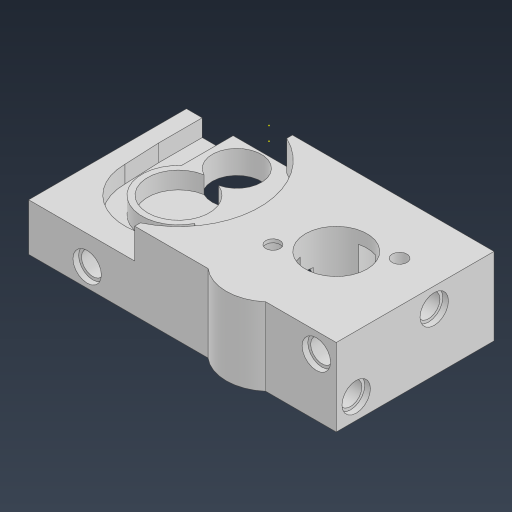
# Autodesk Inventor part: gearbox-holder-left
Saved by Autodesk Inventor 2023 (Build 270158000, 158)
## iProperties
Created: 2025-04-08
Part Number: gearbox-holder-left
Material: Generic
Document SubType Name: Modeling
Designer: szymo
Density: 1 g/cm^3
Appearance: Default
Mass: 8.72272 g
Surface Area: 68.6198 cm^2
Volume: 8.72272 cm^3
Author: szymo
Autodesk Inventor part; units mm, degrees
(part 1 of 2)
ref_plane "YZ Plane" through (0, 0, 0) normal (1, 0, 0) x (0, 1, 0)
ref_plane "XZ Plane" through (0, 0, 0) normal (0, 1, 0) x (-1, 0, 0)
ref_plane "XY Plane" through (0, 0, 0) normal (0, 0, 1) x (1, 0, 0)
ref_plane "Work Plane3" through (-21, -16.2, 14.3) normal (0, 1, 0) x (-1, 0, 0)
sketch "Sketch1" plane through (-21, -16.2, 14.3) normal (0, 1, 0) x (-1, 0, 0)
  circle A0 centre (-40.0468, 4.0664) radius 1.0564 projected
  circle A1 centre (-53.2532, -4.9664) radius 1.0564 projected
  circle A2 centre (-46.65, -0.45) radius 5 projected
  circle A3 centre (-46.65, -0.45) radius 13.85 projected
  line L0 (-23.5981, 5.436) -> (-26.6956, 8.0504) projected
  arc A4 (-26.6956, 8.0504) -> (-28.6306, 5.7578) centre (-18.95, -0.45) ccw projected
  line L1 (-28.6306, 5.7578) -> (-25.5331, 3.1435) projected
  arc A5 (-23.5981, 5.436) -> (-25.5331, 3.1435) centre (-18.95, -0.45) ccw projected
  arc A6 (-11.2044, -8.9504) -> (-9.2694, -6.6578) centre (-18.95, -0.45) ccw projected
  line L2 (-9.2694, -6.6578) -> (-12.3669, -4.0435) projected
  arc A7 (-14.3019, -6.336) -> (-12.3669, -4.0435) centre (-18.95, -0.45) ccw projected
  line L3 (-14.3019, -6.336) -> (-11.2044, -8.9504) projected
  circle A8 centre (-18.95, -0.45) radius 5 projected
  circle A9 centre (-18.95, -0.45) radius 13.85 projected
  line L4 (-25.1095, 12.4) -> (-25.1095, 13.4)
  line L5 (-25.1095, 13.4) -> (-60.5, 13.4)
  line L6 (-60.5, 13.4) -> (-60.5, -14.3)
  line L7 (-60.5, -14.3) -> (-25.1095, -14.3)
  line L8 (-25.1095, -14.3) -> (-25.1095, -13.3)
  circle A10 centre (-18.95, -0.45) radius 14.25
  circle A11 centre (-46.65, -0.45) radius 5.4
  circle A12 centre (-43.0585, 7.5289) radius 1.25 projected
  arc A13 (-39.3343, 3.3134) -> (-38.2806, 2.7608) centre (-36.6798, 7.0946) ccw projected
  arc A14 (-39.6063, 3.0878) -> (-39.3343, 3.3134) centre (-43.0585, 7.5289) ccw projected
  arc A15 (-39.2587, 1.95) -> (-39.6063, 3.0878) centre (-43.8141, 1.1803) ccw projected
  arc A16 (-39.6165, 1.7224) -> (-39.2587, 1.95) centre (-43.0585, 7.5289) ccw projected
  arc A17 (-40.4997, 2.5196) -> (-39.6165, 1.7224) centre (-36.9882, 5.5219) ccw projected
  arc A18 (-40.8192, 2.3688) -> (-40.4997, 2.5196) centre (-43.0585, 7.5289) ccw projected
  arc A19 (-40.7655, 1.1803) -> (-40.8192, 2.3688) centre (-45.3692, 1.5677) ccw projected
  arc A20 (-41.1687, 1.0489) -> (-40.7655, 1.1803) centre (-43.0585, 7.5289) ccw projected
  arc A21 (-41.8258, 2.0407) -> (-41.1687, 1.0489) centre (-37.6781, 4.0753) ccw projected
  arc A22 (-42.1729, 1.9741) -> (-41.8258, 2.0407) centre (-43.0585, 7.5289) ccw projected
  arc A23 (-42.4164, 0.8095) -> (-42.1729, 1.9741) centre (-46.7791, 2.3296) ccw projected
  arc A24 (-42.8396, 0.7825) -> (-42.4164, 0.8095) centre (-43.0585, 7.5289) ccw projected
  arc A25 (-43.2294, 1.9065) -> (-42.8396, 0.7825) centre (-38.706, 2.8458) ccw projected
  arc A26 (-43.5821, 1.9284) -> (-43.2294, 1.9065) centre (-43.0585, 7.5289) ccw projected
  arc A27 (-44.1076, 0.861) -> (-43.5821, 1.9284) centre (-47.9552, 3.4182) ccw projected
  arc A28 (-44.5242, 0.94) -> (-44.1076, 0.861) centre (-43.0585, 7.5289) ccw projected
  arc A29 (-44.6223, 2.1257) -> (-44.5242, 0.94) centre (-40.0074, 1.9105) ccw projected
  arc A30 (-44.9585, 2.2345) -> (-44.6223, 2.1257) centre (-43.0585, 7.5289) ccw projected
  arc A31 (-45.7329, 1.3314) -> (-44.9585, 2.2345) centre (-48.8237, 4.7651) ccw projected
  arc A32 (-46.1168, 1.5115) -> (-45.7329, 1.3314) centre (-43.0585, 7.5289) ccw projected
  arc A33 (-45.9169, 2.6843) -> (-46.1168, 1.5115) centre (-41.5005, 1.3282) ccw projected
  arc A34 (-46.2154, 2.8734) -> (-45.9169, 2.6843) centre (-43.0585, 7.5289) ccw projected
  arc A35 (-47.1901, 2.1912) -> (-46.2154, 2.8734) centre (-49.3299, 6.2857) ccw projected
  arc A36 (-47.5172, 2.4611) -> (-47.1901, 2.1912) centre (-43.0585, 7.5289) ccw projected
  arc A37 (-47.0319, 3.5474) -> (-47.5172, 2.4611) centre (-43.0915, 1.1356) ccw projected
  arc A38 (-47.274, 3.8048) -> (-47.0319, 3.5474) centre (-43.0585, 7.5289) ccw projected
  arc A39 (-48.3878, 3.3864) -> (-47.274, 3.8048) centre (-49.442, 7.8844) ccw projected
  arc A40 (-48.6374, 3.7292) -> (-48.3878, 3.3864) centre (-43.0585, 7.5289) ccw projected
  arc A41 (-47.8972, 4.6606) -> (-48.6374, 3.7292) centre (-44.6804, 1.3446) ccw projected
  arc A42 (-48.0678, 4.9701) -> (-47.8972, 4.6606) centre (-43.0585, 7.5289) ccw projected
  arc A43 (-49.2506, 4.8419) -> (-48.0678, 4.9701) centre (-49.1531, 9.4608) ccw projected
  arc A44 (-49.4071, 5.236) -> (-49.2506, 4.8419) centre (-43.0585, 7.5289) ccw projected
  arc A45 (-48.4585, 5.9541) -> (-49.4071, 5.236) centre (-46.1674, 1.9423) ccw projected
  arc A46 (-48.5467, 6.2963) -> (-48.4585, 5.9541) centre (-43.0585, 7.5289) ccw projected
  arc A47 (-49.7243, 6.4662) -> (-48.5467, 6.2963) centre (-48.4812, 10.9157) ccw projected
  arc A48 (-49.7779, 6.8868) -> (-49.7243, 6.4662) centre (-43.0585, 7.5289) ccw projected
  arc A49 (-48.6805, 7.3465) -> (-49.7779, 6.8868) centre (-47.4591, 2.891) ccw projected
  arc A50 (-48.6809, 7.6999) -> (-48.6805, 7.3465) centre (-43.0585, 7.5289) ccw projected
  arc A51 (-49.7792, 8.1573) -> (-48.6809, 7.6999) centre (-47.4685, 12.1579) ccw projected
  arc A52 (-49.7264, 8.5781) -> (-49.7792, 8.1573) centre (-43.0585, 7.5289) ccw projected
  arc A53 (-48.5493, 8.7504) -> (-49.7264, 8.5781) centre (-48.4743, 4.1311) ccw projected
  arc A54 (-48.4617, 9.0927) -> (-48.5493, 8.7504) centre (-43.0585, 7.5289) ccw projected
  arc A55 (-49.4117, 9.8089) -> (-48.4617, 9.0927) centre (-46.1788, 13.1092) ccw projected
  arc A56 (-49.256, 10.2034) -> (-49.4117, 9.8089) centre (-43.0585, 7.5289) ccw projected
  arc A57 (-48.073, 10.0775) -> (-49.256, 10.2034) centre (-49.1491, 5.5847) ccw projected
  arc A58 (-47.9031, 10.3873) -> (-48.073, 10.0775) centre (-43.0585, 7.5289) ccw projected
  arc A59 (-48.6451, 11.3173) -> (-47.9031, 10.3873) centre (-44.693, 13.7099) ccw projected
  arc A60 (-48.3962, 11.6606) -> (-48.6451, 11.3173) centre (-43.0585, 7.5289) ccw projected
  arc A61 (-47.2816, 11.2445) -> (-48.3962, 11.6606) centre (-49.4413, 7.1604) ccw projected
  arc A62 (-47.04, 11.5023) -> (-47.2816, 11.2445) centre (-43.0585, 7.5289) ccw projected
  arc A63 (-47.5275, 12.5876) -> (-47.04, 11.5023) centre (-43.1045, 13.9222) ccw projected
  arc A64 (-47.201, 12.8583) -> (-47.5275, 12.5876) centre (-43.0585, 7.5289) ccw projected
  arc A65 (-46.2249, 12.178) -> (-47.201, 12.8583) centre (-49.3324, 8.7593) ccw projected
  arc A66 (-45.9268, 12.3677) -> (-46.2249, 12.178) centre (-43.0585, 7.5289) ccw projected
  arc A67 (-46.129, 13.5401) -> (-45.9268, 12.3677) centre (-41.5131, 13.7328) ccw projected
  arc A68 (-45.7455, 13.721) -> (-46.129, 13.5401) centre (-43.0585, 7.5289) ccw projected
  arc A69 (-44.9693, 12.8194) -> (-45.7455, 13.721) centre (-48.8293, 10.281) ccw projected
  arc A70 (-44.6333, 12.929) -> (-44.9693, 12.8194) centre (-43.0585, 7.5289) ccw projected
  arc A71 (-44.5377, 14.1149) -> (-44.6333, 12.929) centre (-40.0188, 13.1536) ccw projected
  arc A72 (-44.1212, 14.1948) -> (-44.5377, 14.1149) centre (-43.0585, 7.5289) ccw projected
  arc A73 (-43.5935, 13.1284) -> (-44.1212, 14.1948) centre (-47.9636, 11.6296) ccw projected
  arc A74 (-43.2409, 13.151) -> (-43.5935, 13.1284) centre (-43.0585, 7.5289) ccw projected
  arc A75 (-42.8533, 14.2758) -> (-43.2409, 13.151) centre (-38.7155, 12.221) ccw projected
  arc A76 (-42.4301, 14.2496) -> (-42.8533, 14.2758) centre (-43.0585, 7.5289) ccw projected
  arc A77 (-42.1842, 13.0856) -> (-42.4301, 14.2496) centre (-46.7897, 12.7207) ccw projected
  arc A78 (-41.837, 13.0197) -> (-42.1842, 13.0856) centre (-43.0585, 7.5289) ccw projected
  arc A79 (-41.1819, 14.0128) -> (-41.837, 13.0197) centre (-37.6851, 10.9935) ccw projected
  arc A80 (-40.7785, 13.8822) -> (-41.1819, 14.0128) centre (-43.0585, 7.5289) ccw projected
  arc A81 (-40.8298, 12.6936) -> (-40.7785, 13.8822) centre (-45.3813, 13.4855) ccw projected
  arc A82 (-40.5099, 12.5435) -> (-40.8298, 12.6936) centre (-43.0585, 7.5289) ccw projected
  arc A83 (-39.6284, 13.3424) -> (-40.5099, 12.5435) centre (-36.9923, 9.5484) ccw projected
  arc A84 (-39.2701, 13.1156) -> (-39.6284, 13.3424) centre (-43.0585, 7.5289) ccw projected
  arc A85 (-39.6154, 11.9771) -> (-39.2701, 13.1156) centre (-43.827, 13.876) ccw projected
  arc A86 (-39.3429, 11.7521) -> (-39.6154, 11.9771) centre (-43.0585, 7.5289) ccw projected
  arc A87 (-38.2904, 12.3068) -> (-39.3429, 11.7521) centre (-36.6807, 7.9763) ccw projected
  arc A88 (-37.9998, 11.998) -> (-38.2904, 12.3068) centre (-43.0585, 7.5289) ccw projected
  arc A89 (-38.6174, 10.9811) -> (-37.9998, 11.998) centre (-42.2244, 13.8678) ccw projected
  arc A90 (-38.4094, 10.6954) -> (-38.6174, 10.9811) centre (-43.0585, 7.5289) ccw projected
  arc A91 (-37.252, 10.9709) -> (-38.4094, 10.6954) centre (-36.7698, 6.3762) ccw projected
  arc A92 (-37.0473, 10.5995) -> (-37.252, 10.9709) centre (-43.0585, 7.5289) ccw projected
  arc A93 (-37.8984, 9.7682) -> (-37.0473, 10.5995) centre (-40.6742, 13.4612) ccw projected
  arc A94 (-37.768, 9.4397) -> (-37.8984, 9.7682) centre (-43.0585, 7.5289) ccw projected
  arc A95 (-36.5784, 9.4187) -> (-37.768, 9.4397) centre (-37.254, 4.8485) ccw projected
  arc A96 (-36.4725, 9.0081) -> (-36.5784, 9.4187) centre (-43.0585, 7.5289) ccw projected
  arc A97 (-37.5036, 8.4146) -> (-36.4725, 9.0081) centre (-39.2738, 12.6819) ccw projected
  arc A98 (-37.459, 8.064) -> (-37.5036, 8.4146) centre (-43.0585, 7.5289) ccw projected
  arc A99 (-36.312, 7.7478) -> (-37.459, 8.064) centre (-38.103, 3.4892) ccw projected
  arc A100 (-36.3116, 7.3238) -> (-36.312, 7.7478) centre (-43.0585, 7.5289) ccw projected
  arc A101 (-37.4579, 7.0053) -> (-36.3116, 7.3238) centre (-38.1113, 11.5788) ccw projected
  arc A102 (-37.5018, 6.6547) -> (-37.4579, 7.0053) centre (-43.0585, 7.5289) ccw projected
  arc A103 (-36.4695, 6.0632) -> (-37.5018, 6.6547) centre (-39.2633, 2.3837) ccw projected
  arc A104 (-36.5746, 5.6524) -> (-36.4695, 6.0632) centre (-43.0585, 7.5289) ccw projected
  arc A105 (-37.7641, 5.6289) -> (-36.5746, 5.6524) centre (-37.2595, 10.2212) ccw projected
  arc A106 (-37.8938, 5.3003) -> (-37.7641, 5.6289) centre (-43.0585, 7.5289) ccw projected
  arc A107 (-37.0411, 4.4706) -> (-37.8938, 5.3003) centre (-40.6621, 1.6016) ccw projected
  arc A108 (-37.245, 4.0988) -> (-37.0411, 4.4706) centre (-43.0585, 7.5289) ccw projected
  arc A109 (-38.4029, 4.372) -> (-37.245, 4.0988) centre (-36.7722, 8.6945) ccw projected
  arc A110 (-38.6103, 4.0859) -> (-38.4029, 4.372) centre (-43.0585, 7.5289) ccw projected
  arc A111 (-37.9907, 3.0703) -> (-38.6103, 4.0859) centre (-42.2115, 1.1918) ccw projected
  arc A112 (-38.2806, 2.7608) -> (-37.9907, 3.0703) centre (-43.0585, 7.5289) ccw projected
  circle A113 centre (-43.0585, 7.5289) radius 6.75
  circle A114 centre (-43.0585, 7.5289) radius 7.15
  circle A115 centre (-43.0585, 7.5289) radius 7.75
  point P0 (-21, -14.3)
  point P1 (-37.9995, 13.4)
  point P2 (-48.1174, 13.4)
  dimension "d2" = 0.4
  dimension "d3" = 1
  dimension "d5" = 1
  dimension "d6" = 0.4
  dimension "d13" = 0.4
  dimension "d14" = 0.6
  constraints: 10 end point, 4 centre point, 4 perpendicular, 3 tangent, 2 point on circle, 1 coincident, 1 vertical, 3 other
  measures "d2" radial gap between concentric circles of A9 A10
  measures "d3" distance of L7.end L8.end
  measures "d5" distance of L4.start L4.end
  measures "d6" radial gap between concentric circles of A2 A11
  measures "d14" radial gap between concentric circles of A114 A115
extrude "Extrusion1" add sketch "Sketch1" against normal blind 3.1 contours A0 A13 A14 | A0 A14 A15 A16 A17 A18 A19 A20 A21 A22 A11 A42 A43 A44 A45 A46 A47 A48 A49 A50 A51 A52 A53 A54 A55 A56 A57 A58 A59 A60 A61 A62 A63 A64 A65 A66 A67 A3 A69 A70 A71 A93 A94 A95 A97 A98 A99 A100 A101 A102 A103 A104 A105 A106 A107 A108 A109 A110 A111 A112 A13 | A14 A13 A0 | A0 A13 A113 A15 A14 | A112 A113 A108 A104 A100 A3 A114 A11 A20 A16 | A111 A110 A109 A113 | A113 A19 A18 A17 | A107 A106 A105 A113 | A113 A11 A22 A21 | A103 A102 A101 A113 | A114 A3 A115 A11 | A11 A113 A43 A42 | A115 A3 A10 A11 | A11 A114 A3 A113 A64 A60 A56 A52 A48 A44 | A115 L5 L4 A10 A3 | A3 A114 L5 A115 | A3 A113 A96 A92 A88 A84 L5 A114 | A99 A98 A97 A3 A113 | A11 A115 A3 A114 | A3 A97 A113 | A114 L5 A115 | L5 A113 A80 A76 A72 A68 A3 A114 | A114 L5 A3 | A3 A115 L5 A114 | A113 A47 A46 A45 | A3 L6 L5 A115 | A10 L8 L7 A3 | A3 A95 A96 A97 | A113 A83 A82 A81 L5 | L5 A81 A113 | A3 L7 L6 | A95 A94 A93 A3 | A3 A93 A113 A95 | A81 A82 A83 A84 A85 A86 A87 A88 A89 A90 A91 A92 A93 A3 A71 L5 A73 A74 A75 A77 A78 A79 | L5 A79 A80 A81 | L5 A67 A3 | A113 A67 L5 | A3 A67 A66 A65 A113 | A113 A51 A50 A49 | A79 A78 A77 L5 | L5 A77 A113 A79 | A113 A87 A86 A85 | A67 L5 A69 A3 | A67 A68 A69 L5 | A71 A70 A69 A3 | A3 A69 L5 A71 | A91 A90 A89 A113 | L5 A75 A76 A77 | A69 A113 A71 L5 | A63 A62 A61 A113 | A113 A55 A54 A53 | A71 A72 A73 L5 | A75 A74 A73 L5 | L5 A73 A113 A75 | A59 A58 A57 A113 | A1 | A12
sketch "Sketch2" plane through (-21, -19.3, 14.3) normal (0, -1, 0) x (1, 0, 0)
  circle A0 centre (43.0585, 7.5289) radius 1.25 projected
  arc A1 (38.2806, 2.7608) -> (39.3343, 3.3134) centre (36.6798, 7.0946) ccw projected
  arc A2 (39.3343, 3.3134) -> (39.6063, 3.0878) centre (43.0585, 7.5289) ccw projected
  arc A3 (39.6063, 3.0878) -> (39.2587, 1.95) centre (43.8141, 1.1803) ccw projected
  arc A4 (39.2587, 1.95) -> (39.6165, 1.7224) centre (43.0585, 7.5289) ccw projected
  arc A5 (39.6165, 1.7224) -> (40.4997, 2.5196) centre (36.9882, 5.5219) ccw projected
  arc A6 (40.4997, 2.5196) -> (40.8192, 2.3688) centre (43.0585, 7.5289) ccw projected
  arc A7 (40.8192, 2.3688) -> (40.7655, 1.1803) centre (45.3692, 1.5677) ccw projected
  arc A8 (40.7655, 1.1803) -> (41.1687, 1.0489) centre (43.0585, 7.5289) ccw projected
  arc A9 (41.1687, 1.0489) -> (41.8258, 2.0407) centre (37.6781, 4.0753) ccw projected
  arc A10 (41.8258, 2.0407) -> (42.1729, 1.9741) centre (43.0585, 7.5289) ccw projected
  arc A11 (42.1729, 1.9741) -> (42.4164, 0.8095) centre (46.7791, 2.3296) ccw projected
  arc A12 (42.4164, 0.8095) -> (42.8396, 0.7825) centre (43.0585, 7.5289) ccw projected
  arc A13 (42.8396, 0.7825) -> (43.2294, 1.9065) centre (38.706, 2.8458) ccw projected
  arc A14 (43.2294, 1.9065) -> (43.5821, 1.9284) centre (43.0585, 7.5289) ccw projected
  arc A15 (43.5821, 1.9284) -> (44.1076, 0.861) centre (47.9552, 3.4182) ccw projected
  arc A16 (44.1076, 0.861) -> (44.5242, 0.94) centre (43.0585, 7.5289) ccw projected
  arc A17 (44.5242, 0.94) -> (44.6223, 2.1257) centre (40.0074, 1.9105) ccw projected
  arc A18 (44.6223, 2.1257) -> (44.9585, 2.2345) centre (43.0585, 7.5289) ccw projected
  arc A19 (44.9585, 2.2345) -> (45.7329, 1.3314) centre (48.8237, 4.7651) ccw projected
  arc A20 (45.7329, 1.3314) -> (46.1168, 1.5115) centre (43.0585, 7.5289) ccw projected
  arc A21 (46.1168, 1.5115) -> (45.9169, 2.6843) centre (41.5005, 1.3282) ccw projected
  arc A22 (45.9169, 2.6843) -> (46.2154, 2.8734) centre (43.0585, 7.5289) ccw projected
  arc A23 (46.2154, 2.8734) -> (47.1901, 2.1912) centre (49.3299, 6.2857) ccw projected
  arc A24 (47.1901, 2.1912) -> (47.5172, 2.4611) centre (43.0585, 7.5289) ccw projected
  arc A25 (47.5172, 2.4611) -> (47.0319, 3.5474) centre (43.0915, 1.1356) ccw projected
  arc A26 (47.0319, 3.5474) -> (47.274, 3.8048) centre (43.0585, 7.5289) ccw projected
  arc A27 (47.274, 3.8048) -> (48.3878, 3.3864) centre (49.442, 7.8844) ccw projected
  arc A28 (48.3878, 3.3864) -> (48.6374, 3.7292) centre (43.0585, 7.5289) ccw projected
  arc A29 (48.6374, 3.7292) -> (47.8972, 4.6606) centre (44.6804, 1.3446) ccw projected
  arc A30 (47.8972, 4.6606) -> (48.0678, 4.9701) centre (43.0585, 7.5289) ccw projected
  arc A31 (48.0678, 4.9701) -> (49.2506, 4.8419) centre (49.1531, 9.4608) ccw projected
  arc A32 (49.2506, 4.8419) -> (49.4071, 5.236) centre (43.0585, 7.5289) ccw projected
  arc A33 (49.4071, 5.236) -> (48.4585, 5.9541) centre (46.1674, 1.9423) ccw projected
  arc A34 (48.4585, 5.9541) -> (48.5467, 6.2963) centre (43.0585, 7.5289) ccw projected
  arc A35 (48.5467, 6.2963) -> (49.7243, 6.4662) centre (48.4812, 10.9157) ccw projected
  arc A36 (49.7243, 6.4662) -> (49.7779, 6.8868) centre (43.0585, 7.5289) ccw projected
  arc A37 (49.7779, 6.8868) -> (48.6805, 7.3465) centre (47.4591, 2.891) ccw projected
  arc A38 (48.6805, 7.3465) -> (48.6809, 7.6999) centre (43.0585, 7.5289) ccw projected
  arc A39 (48.6809, 7.6999) -> (49.7792, 8.1573) centre (47.4685, 12.1579) ccw projected
  arc A40 (49.7792, 8.1573) -> (49.7264, 8.5781) centre (43.0585, 7.5289) ccw projected
  arc A41 (49.7264, 8.5781) -> (48.5493, 8.7504) centre (48.4743, 4.1311) ccw projected
  arc A42 (48.5493, 8.7504) -> (48.4617, 9.0927) centre (43.0585, 7.5289) ccw projected
  arc A43 (48.4617, 9.0927) -> (49.4117, 9.8089) centre (46.1788, 13.1092) ccw projected
  arc A44 (49.4117, 9.8089) -> (49.256, 10.2034) centre (43.0585, 7.5289) ccw projected
  arc A45 (49.256, 10.2034) -> (48.073, 10.0775) centre (49.1491, 5.5847) ccw projected
  arc A46 (48.073, 10.0775) -> (47.9031, 10.3873) centre (43.0585, 7.5289) ccw projected
  arc A47 (47.9031, 10.3873) -> (48.6451, 11.3173) centre (44.693, 13.7099) ccw projected
  arc A48 (48.6451, 11.3173) -> (48.3962, 11.6606) centre (43.0585, 7.5289) ccw projected
  arc A49 (48.3962, 11.6606) -> (47.2816, 11.2445) centre (49.4413, 7.1604) ccw projected
  arc A50 (47.2816, 11.2445) -> (47.04, 11.5023) centre (43.0585, 7.5289) ccw projected
  arc A51 (47.04, 11.5023) -> (47.5275, 12.5876) centre (43.1045, 13.9222) ccw projected
  arc A52 (47.5275, 12.5876) -> (47.201, 12.8583) centre (43.0585, 7.5289) ccw projected
  arc A53 (47.201, 12.8583) -> (46.2249, 12.178) centre (49.3324, 8.7593) ccw projected
  arc A54 (46.2249, 12.178) -> (45.9268, 12.3677) centre (43.0585, 7.5289) ccw projected
  arc A55 (45.9268, 12.3677) -> (46.129, 13.5401) centre (41.5131, 13.7328) ccw projected
  arc A56 (46.129, 13.5401) -> (45.7455, 13.721) centre (43.0585, 7.5289) ccw projected
  arc A57 (45.7455, 13.721) -> (44.9693, 12.8194) centre (48.8293, 10.281) ccw projected
  arc A58 (44.9693, 12.8194) -> (44.6333, 12.929) centre (43.0585, 7.5289) ccw projected
  arc A59 (44.6333, 12.929) -> (44.5377, 14.1149) centre (40.0188, 13.1536) ccw projected
  arc A60 (44.5377, 14.1149) -> (44.1212, 14.1948) centre (43.0585, 7.5289) ccw projected
  arc A61 (44.1212, 14.1948) -> (43.5935, 13.1284) centre (47.9636, 11.6296) ccw projected
  arc A62 (43.5935, 13.1284) -> (43.2409, 13.151) centre (43.0585, 7.5289) ccw projected
  arc A63 (43.2409, 13.151) -> (42.8533, 14.2758) centre (38.7155, 12.221) ccw projected
  arc A64 (42.8533, 14.2758) -> (42.4301, 14.2496) centre (43.0585, 7.5289) ccw projected
  arc A65 (42.4301, 14.2496) -> (42.1842, 13.0856) centre (46.7897, 12.7207) ccw projected
  arc A66 (42.1842, 13.0856) -> (41.837, 13.0197) centre (43.0585, 7.5289) ccw projected
  arc A67 (41.837, 13.0197) -> (41.1819, 14.0128) centre (37.6851, 10.9935) ccw projected
  arc A68 (41.1819, 14.0128) -> (40.7785, 13.8822) centre (43.0585, 7.5289) ccw projected
  arc A69 (40.7785, 13.8822) -> (40.8298, 12.6936) centre (45.3813, 13.4855) ccw projected
  arc A70 (40.8298, 12.6936) -> (40.5099, 12.5435) centre (43.0585, 7.5289) ccw projected
  arc A71 (40.5099, 12.5435) -> (39.6284, 13.3424) centre (36.9923, 9.5484) ccw projected
  arc A72 (39.6284, 13.3424) -> (39.2701, 13.1156) centre (43.0585, 7.5289) ccw projected
  arc A73 (39.2701, 13.1156) -> (39.6154, 11.9771) centre (43.827, 13.876) ccw projected
  arc A74 (39.6154, 11.9771) -> (39.3429, 11.7521) centre (43.0585, 7.5289) ccw projected
  arc A75 (39.3429, 11.7521) -> (38.2904, 12.3068) centre (36.6807, 7.9763) ccw projected
  arc A76 (38.2904, 12.3068) -> (37.9998, 11.998) centre (43.0585, 7.5289) ccw projected
  arc A77 (37.9998, 11.998) -> (38.6174, 10.9811) centre (42.2244, 13.8678) ccw projected
  arc A78 (38.6174, 10.9811) -> (38.4094, 10.6954) centre (43.0585, 7.5289) ccw projected
  arc A79 (38.4094, 10.6954) -> (37.252, 10.9709) centre (36.7698, 6.3762) ccw projected
  arc A80 (37.252, 10.9709) -> (37.0473, 10.5995) centre (43.0585, 7.5289) ccw projected
  arc A81 (37.0473, 10.5995) -> (37.8984, 9.7682) centre (40.6742, 13.4612) ccw projected
  arc A82 (37.8984, 9.7682) -> (37.768, 9.4397) centre (43.0585, 7.5289) ccw projected
  arc A83 (37.768, 9.4397) -> (36.5784, 9.4187) centre (37.254, 4.8485) ccw projected
  arc A84 (36.5784, 9.4187) -> (36.4725, 9.0081) centre (43.0585, 7.5289) ccw projected
  arc A85 (36.4725, 9.0081) -> (37.5036, 8.4146) centre (39.2738, 12.6819) ccw projected
  arc A86 (37.5036, 8.4146) -> (37.459, 8.064) centre (43.0585, 7.5289) ccw projected
  arc A87 (37.459, 8.064) -> (36.312, 7.7478) centre (38.103, 3.4892) ccw projected
  arc A88 (36.312, 7.7478) -> (36.3116, 7.3238) centre (43.0585, 7.5289) ccw projected
  arc A89 (36.3116, 7.3238) -> (37.4579, 7.0053) centre (38.1113, 11.5788) ccw projected
  arc A90 (37.4579, 7.0053) -> (37.5018, 6.6547) centre (43.0585, 7.5289) ccw projected
  arc A91 (37.5018, 6.6547) -> (36.4695, 6.0632) centre (39.2633, 2.3837) ccw projected
  arc A92 (36.4695, 6.0632) -> (36.5746, 5.6524) centre (43.0585, 7.5289) ccw projected
  arc A93 (36.5746, 5.6524) -> (37.7641, 5.6289) centre (37.2595, 10.2212) ccw projected
  arc A94 (37.7641, 5.6289) -> (37.8938, 5.3003) centre (43.0585, 7.5289) ccw projected
  arc A95 (37.8938, 5.3003) -> (37.0411, 4.4706) centre (40.6621, 1.6016) ccw projected
  arc A96 (37.0411, 4.4706) -> (37.245, 4.0988) centre (43.0585, 7.5289) ccw projected
  arc A97 (37.245, 4.0988) -> (38.4029, 4.372) centre (36.7722, 8.6945) ccw projected
  arc A98 (38.4029, 4.372) -> (38.6103, 4.0859) centre (43.0585, 7.5289) ccw projected
  arc A99 (38.6103, 4.0859) -> (37.9907, 3.0703) centre (42.2115, 1.1918) ccw projected
  arc A100 (37.9907, 3.0703) -> (38.2806, 2.7608) centre (43.0585, 7.5289) ccw projected
  circle A101 centre (43.0585, 7.5289) radius 6.75
  circle A102 centre (43.0585, 7.5289) radius 7.15
  circle A103 centre (43.0585, 7.5289) radius 7.75
  line L0 (25.1095, 13.4) -> (25.1095, 12.4) projected
  arc A104 (25.1095, -13.3) -> (25.1095, 12.4) centre (18.95, -0.45) ccw projected
  line L1 (25.1095, -13.3) -> (25.1095, -14.3) projected
  line L2 (25.1095, -14.3) -> (60.5, -14.3) projected
  line L3 (60.5, -14.3) -> (60.5, 13.4) projected
  line L4 (60.5, 13.4) -> (48.1174, 13.4) projected
  circle A105 centre (46.65, -0.45) radius 5.4 projected
  arc A106 (48.1174, 13.4) -> (37.9995, 13.4) centre (43.0585, 7.5289) ccw projected
  line L5 (37.9995, 13.4) -> (25.1095, 13.4) projected
  point P0 (21, -14.3)
  point P1 (49.3884, 4.2041)
  point P2 (41.3503, 0.586)
  point P3 (37.8284, 13.4)
  point P4 (37.9995, 13.4)
  dimension "d9" = 0.4
  dimension "d10" = 0.6
  constraints: 2 centre point, 1 coincident, 3 other
  measures "d10" radial gap between concentric circles of A102 A103
extrude "Extrusion2" add sketch "Sketch2" along normal blind 2.2 contours A105 A103 A102 | A105 A103 L4 L3 L2 L1 A104 L0 L5 picked at (47.797, 13.0993)
sketch "Sketch3" plane through (-21, -21.5, 14.3) normal (0, -1, 0) x (1, 0, 0)
  line L0 (37.9995, 13.4) -> (25.1095, 13.4) projected
  line L1 (25.1095, 13.4) -> (25.1095, 12.4) projected
  arc A0 (25.1095, -13.3) -> (25.1095, 12.4) centre (18.95, -0.45) ccw projected
  line L2 (25.1095, -13.3) -> (25.1095, -14.3) projected
  line L3 (25.1095, -14.3) -> (60.5, -14.3) projected
  line L4 (60.5, -14.3) -> (60.5, 13.4) projected
  line L5 (60.5, 13.4) -> (48.1174, 13.4) projected
  arc A1 (48.1174, 13.4) -> (37.9995, 13.4) centre (43.0585, 7.5289) ccw projected
  arc A2 (49.3884, 4.2041) -> (41.3503, 0.586) centre (43.0585, 7.5289) ccw projected
  arc A3 (41.3503, 0.586) -> (49.3884, 4.2041) centre (46.65, -0.45) ccw projected
  circle A4 centre (20, -9.6433) radius 12.5 projected
  line L6 (25.1095, 12.4) -> (25.1095, 13.4) projected
  line L7 (25.1095, 13.4) -> (13.5564, 13.4)
  line L8 (13.5564, 13.4) -> (6.5, 13.4)
  line L9 (6.5, 13.4) -> (6.5, -14.3)
  line L10 (25.1095, -14.3) -> (25.1095, -13.3) projected
  line L11 (6.5, -14.3) -> (25.1095, -14.3)
  line L12 (6.5, 13.4) -> (12.5, 13.4)
  line L13 (12.5, 13.4) -> (12.5, 7.4)
  line L14 (12.5, 7.4) -> (6.5, 7.4)
  line L15 (6.5, 7.4) -> (6.5, 13.4)
  circle A5 centre (18.95, -0.45) radius 5.4
  circle A6 centre (18.95, -0.45) radius 6.4
  circle A7 centre (20, -9.6433) radius 4 projected
  circle A8 centre (20, -9.6433) radius 4.3
  circle A9 centre (20, -9.6433) radius 5.3
  line L16 (23.5981, 5.436) -> (26.6956, 8.0504) projected
  arc A10 (28.6306, 5.7578) -> (26.6956, 8.0504) centre (18.95, -0.45) ccw projected
  line L17 (28.6306, 5.7578) -> (25.5331, 3.1435) projected
  arc A11 (25.5331, 3.1435) -> (23.5981, 5.436) centre (18.95, -0.45) ccw projected
  arc A12 (9.2694, -6.6578) -> (11.2044, -8.9504) centre (18.95, -0.45) ccw projected
  line L18 (9.2694, -6.6578) -> (12.3669, -4.0435) projected
  arc A13 (12.3669, -4.0435) -> (14.3019, -6.336) centre (18.95, -0.45) ccw projected
  line L19 (14.3019, -6.336) -> (11.2044, -8.9504) projected
  circle A14 centre (18.95, -0.45) radius 5 projected
  circle A15 centre (18.95, -0.45) radius 13.85 projected
  line L20 (14.7, -5.2351) -> (14.7, -14.3)
  line L21 (9.2694, -6.6578) -> (9.2694, -14.3)
  circle A16 centre (18.95, -0.45) radius 9.4
  line L22 (26.6956, 8.0504) -> (20.7823, 8.7697)
  line L23 (9.55, -0.45) -> (9.2694, -6.6578)
  line L24 (25.5331, 3.1435) -> (24.6721, 2.4167)
  point P0 (21, -14.3)
  point P1 (15.3858, -7.0359)
  point P2 (12.5, 13.4)
  point P3 (13.1701, -14.3)
  point P4 (8.7954, -14.3)
  point P5 (20.9759, -5.4556)
  point P6 (18.1049, -5.7835)
  dimension "d16" = 6
  dimension "d17" = 6
  dimension "d18" = 13.5
  dimension "d34" = 1
  dimension "d37" = 0.3
  dimension "d141" = 1
  dimension "d142" = 0.4
  dimension "d144" = 3
  constraints: 26 end point, 5 perpendicular, 4 centre point, 4 point on circle, 4 point on line, 2 coincident, 2 collinear, 2 horizontal, 2 parallel, 1 vertical, 3 other
  measures "d16" distance of L13.end L14.end
  measures "d17" distance of L12.end L13.end
  measures "d18" distance from line of L9 A4.centre
  measures "d34" radial gap between concentric circles of A5 A6
  measures "d37" radial gap between concentric circles of A7 A8
  measures "d142" radial gap between concentric circles of A5 A14
  measures "d144" radial gap between concentric circles of A6 A16
extrude "Extrusion3" add sketch "Sketch3" along normal blind 0.4 contours A1 L5 L4 L3 A4 A0 L1 L0 | L1 A0 A4 A15 L7 | A15 L13 L8 L7 | A15 A4 A16 L17 A10 L22 L23 L9 L14 L13 | A4 L3 L2 A0 | A0 L2 L11 A9 A15 A4 | A15 L14 L9 L8 L13 | L13 L14 A15 | A15 A9 A16 A4 | A15 L9 L14 | A16 A9 A6 A4 | A4 A6 L24 L17 A16 | A15 A9 A16 A8 | A9 L11 A15 | L11 L9 A15 A4 | A4 A15 L21 L11 | A6 A9 A5 A4 | A4 A5 A6 | L11 A9 A15 | A4 L23 L21 A15 | L11 L20 A15 A9 | A16 A8 A6 A9 | A15 L20 A9 | A5 A9 A6 A4 | A6 A8 A5 A9 | L20 A16 A9 | A5 A8 A6 A9 | A6 A9 A16 L20 | A9 A6 A8 A16
sketch "Sketch4" plane through (-21, -21.9, 14.3) normal (0, -1, 0) x (1, 0, 0)
  circle A0 centre (35.7557, 2.709) radius 1.25 projected
  arc A1 (29.263, 4.5551) -> (30.2592, 3.9047) centre (32.2659, 8.066) ccw projected
  arc A2 (30.2592, 3.9047) -> (30.195, 3.5572) centre (35.7557, 2.709) ccw projected
  arc A3 (30.195, 3.5572) -> (29.0321, 3.3058) centre (30.5815, -1.0466) ccw projected
  arc A4 (29.0321, 3.3058) -> (29.0079, 2.8825) centre (35.7557, 2.709) ccw projected
  arc A5 (29.0079, 2.8825) -> (30.1346, 2.5002) centre (31.0433, 7.0299) ccw projected
  arc A6 (30.1346, 2.5002) -> (30.1588, 2.1476) centre (35.7557, 2.709) ccw projected
  arc A7 (30.1588, 2.1476) -> (29.0949, 1.615) centre (31.678, -2.2153) ccw projected
  arc A8 (29.0949, 1.615) -> (29.1768, 1.1989) centre (35.7557, 2.709) ccw projected
  arc A9 (29.1768, 1.1989) -> (30.3631, 1.1088) centre (30.1168, 5.7222) ccw projected
  arc A10 (30.3631, 1.1088) -> (30.4742, 0.7734) centre (35.7557, 2.709) ccw projected
  arc A11 (30.4742, 0.7734) -> (29.5763, -0.0071) centre (33.0308, -3.0747) ccw projected
  arc A12 (29.5763, -0.0071) -> (29.759, -0.3898) centre (35.7557, 2.709) ccw projected
  arc A13 (29.759, -0.3898) -> (30.9304, -0.182) centre (29.5446, 4.2252) ccw projected
  arc A14 (30.9304, -0.182) -> (31.1215, -0.4793) centre (35.7557, 2.709) ccw projected
  arc A15 (31.1215, -0.4793) -> (30.4459, -1.4585) centre (34.5547, -3.5706) ccw projected
  arc A16 (30.4459, -1.4585) -> (30.718, -1.7837) centre (35.7557, 2.709) ccw projected
  arc A17 (30.718, -1.7837) -> (31.801, -1.2911) centre (29.3627, 2.6329) ccw projected
  arc A18 (31.801, -1.2911) -> (32.06, -1.5316) centre (35.7557, 2.709) ccw projected
  arc A19 (32.06, -1.5316) -> (31.6491, -2.6481) centre (36.1542, -3.672) ccw projected
  arc A20 (31.6491, -2.6481) -> (31.9936, -2.8954) centre (35.7557, 2.709) ccw projected
  arc A21 (31.9936, -2.8954) -> (32.92, -2.149) centre (29.5824, 1.0455) ccw projected
  arc A22 (32.92, -2.149) -> (33.2307, -2.3174) centre (35.7557, 2.709) ccw projected
  arc A23 (33.2307, -2.3174) -> (33.1104, -3.5011) centre (37.7285, -3.3724) ccw projected
  arc A24 (33.1104, -3.5011) -> (33.5055, -3.6549) centre (35.7557, 2.709) ccw projected
  arc A25 (33.5055, -3.6549) -> (34.2173, -2.7015) centre (30.1901, -0.4375) ccw projected
  arc A26 (34.2173, -2.7015) -> (34.56, -2.7874) centre (35.7557, 2.709) ccw projected
  arc A27 (34.56, -2.7874) -> (34.7379, -3.9638) centre (39.1789, -2.6908) ccw projected
  arc A28 (34.7379, -3.9638) -> (35.1589, -4.0146) centre (35.7557, 2.709) ccw projected
  arc A29 (35.1589, -4.0146) -> (35.6111, -2.9141) centre (31.1475, -1.7228) ccw projected
  arc A30 (35.6111, -2.9141) -> (35.9645, -2.9121) centre (35.7557, 2.709) ccw projected
  arc A31 (35.9645, -2.9121) -> (36.4293, -4.0073) centre (40.4143, -1.6698) ccw projected
  arc A32 (36.4293, -4.0073) -> (36.8497, -3.9517) centre (35.7557, 2.709) ccw projected
  arc A33 (36.8497, -3.9517) -> (37.0141, -2.7734) centre (32.3944, -2.7295) ccw projected
  arc A34 (37.0141, -2.7734) -> (37.3559, -2.6836) centre (35.7557, 2.709) ccw projected
  arc A35 (37.3559, -2.6836) -> (38.0784, -3.6288) centre (41.3569, -0.3737) ccw projected
  arc A36 (38.0784, -3.6288) -> (38.4718, -3.4704) centre (35.7557, 2.709) ccw projected
  arc A37 (38.4718, -3.4704) -> (38.338, -2.2882) centre (33.8525, -3.3946) ccw projected
  arc A38 (38.338, -2.2882) -> (38.6467, -2.1162) centre (35.7557, 2.709) ccw projected
  arc A39 (38.6467, -2.1162) -> (39.5816, -2.852) centre (41.9475, 1.1161) ccw projected
  arc A40 (39.5816, -2.852) -> (39.9232, -2.6008) centre (35.7557, 2.709) ccw projected
  arc A41 (39.9232, -2.6008) -> (39.4996, -1.489) centre (35.4302, -3.6761) ccw projected
  arc A42 (39.4996, -1.489) -> (39.7558, -1.2457) centre (35.7557, 2.709) ccw projected
  arc A43 (39.7558, -1.2457) -> (40.8444, -1.7258) centre (42.1491, 2.706) ccw projected
  arc A44 (40.8444, -1.7258) -> (41.1128, -1.3976) centre (35.7557, 2.709) ccw projected
  arc A45 (41.1128, -1.3976) -> (40.426, -0.4261) centre (37.0283, -3.5565) ccw projected
  arc A46 (40.426, -0.4261) -> (40.6136, -0.1266) centre (35.7557, 2.709) ccw projected
  arc A47 (40.6136, -0.1266) -> (41.7874, -0.321) centre (41.949, 4.2961) ccw projected
  arc A48 (41.7874, -0.321) -> (41.9657, 0.0637) centre (35.7557, 2.709) ccw projected
  arc A49 (41.9657, 0.0637) -> (41.0589, 0.8339) centre (38.5465, -3.0432) ccw projected
  arc A50 (41.0589, 0.8339) -> (41.1662, 1.1706) centre (35.7557, 2.709) ccw projected
  arc A51 (41.1662, 1.1706) -> (42.3514, 1.2742) centre (41.3597, 5.7865) ccw projected
  arc A52 (42.3514, 1.2742) -> (42.4285, 1.6912) centre (35.7557, 2.709) ccw projected
  arc A53 (42.4285, 1.6912) -> (41.3586, 2.2117) centre (39.8893, -2.1684) ccw projected
  arc A54 (41.3586, 2.2117) -> (41.3788, 2.5645) centre (35.7557, 2.709) ccw projected
  arc A55 (41.3788, 2.5645) -> (42.501, 2.9596) centre (40.4183, 7.0835) ccw projected
  arc A56 (42.501, 2.9596) -> (42.472, 3.3827) centre (35.7557, 2.709) ccw projected
  arc A57 (42.472, 3.3827) -> (41.3063, 3.6207) centre (40.9724, -0.9872) ccw projected
  arc A58 (41.3063, 3.6207) -> (41.2381, 3.9674) centre (35.7557, 2.709) ccw projected
  arc A59 (41.2381, 3.9674) -> (42.2268, 4.6292) centre (39.184, 8.1056) ccw projected
  arc A60 (42.2268, 4.6292) -> (42.0934, 5.0318) centre (35.7557, 2.709) ccw projected
  arc A61 (42.0934, 5.0318) -> (40.9052, 4.9724) centre (41.7277, 0.4263) ccw projected
  arc A62 (40.9052, 4.9724) -> (40.7529, 5.2913) centre (35.7557, 2.709) ccw projected
  arc A63 (40.7529, 5.2913) -> (41.5459, 6.1782) centre (37.7342, 8.7886) ccw projected
  arc A64 (41.5459, 6.1782) -> (41.3167, 6.5349) centre (35.7557, 2.709) ccw projected
  arc A65 (41.3167, 6.5349) -> (40.1805, 6.182) centre (42.1078, 1.9832) ccw projected
  arc A66 (40.1805, 6.182) -> (39.9537, 6.453) centre (35.7557, 2.709) ccw projected
  arc A67 (39.9537, 6.453) -> (40.5013, 7.5092) centre (36.1601, 9.0897) ccw projected
  arc A68 (40.5013, 7.5092) -> (40.1905, 7.7977) centre (35.7557, 2.709) ccw projected
  arc A69 (40.1905, 7.7977) -> (39.1778, 7.1733) centre (42.0887, 3.5857) ccw projected
  arc A70 (39.1778, 7.1733) -> (38.8907, 7.3793) centre (35.7557, 2.709) ccw projected
  arc A71 (38.8907, 7.3793) -> (39.1584, 8.5386) centre (34.5606, 8.9898) ccw projected
  arc A72 (39.1584, 8.5386) -> (38.7857, 8.7407) centre (35.7557, 2.709) ccw projected
  arc A73 (38.7857, 8.7407) -> (37.9601, 7.8841) centre (41.6717, 5.1332) ccw projected
  arc A74 (37.9601, 7.8841) -> (37.6308, 8.0123) centre (35.7557, 2.709) ccw projected
  arc A75 (37.6308, 8.0123) -> (37.6018, 9.2017) centre (33.0362, 8.4952) ccw projected
  arc A76 (37.6018, 9.2017) -> (37.1905, 9.3048) centre (35.7557, 2.709) ccw projected
  arc A77 (37.1905, 9.3048) -> (36.6038, 8.2697) centre (40.883, 6.5283) ccw projected
  arc A78 (36.6038, 8.2697) -> (36.253, 8.312) centre (35.7557, 2.709) ccw projected
  arc A79 (36.253, 8.312) -> (35.9291, 9.4568) centre (31.6826, 7.6371) ccw projected
  arc A80 (35.9291, 9.4568) -> (35.5051, 9.4544) centre (35.7557, 2.709) ccw projected
  arc A81 (35.5051, 9.4544) -> (35.1943, 8.3059) centre (39.7721, 7.6834) ccw projected
  arc A82 (35.1943, 8.3059) -> (34.844, 8.2596) centre (35.7557, 2.709) ccw projected
  arc A83 (34.844, 8.2596) -> (34.2456, 9.2879) centre (30.585, 6.4694) ccw projected
  arc A84 (34.2456, 9.2879) -> (33.8355, 9.1801) centre (35.7557, 2.709) ccw projected
  arc A85 (33.8355, 9.1801) -> (33.82, 7.9905) centre (38.4088, 8.526) ccw projected
  arc A86 (33.82, 7.9905) -> (33.4922, 7.8585) centre (35.7557, 2.709) ccw projected
  arc A87 (33.4922, 7.8585) -> (32.6569, 8.7057) centre (29.8123, 5.0654) ccw projected
  arc A88 (32.6569, 8.7057) -> (32.2865, 8.4993) centre (35.7557, 2.709) ccw projected
  arc A89 (32.2865, 8.4993) -> (32.5674, 7.3432) centre (36.8789, 9.003) ccw projected
  arc A90 (32.5674, 7.3432) -> (32.2827, 7.1339) centre (35.7557, 2.709) ccw projected
  arc A91 (32.2827, 7.1339) -> (31.2629, 7.7467) centre (29.413, 3.5133) ccw projected
  arc A92 (31.2629, 7.7467) -> (30.9555, 7.4546) centre (35.7557, 2.709) ccw projected
  arc A93 (30.9555, 7.4546) -> (31.5151, 6.4047) centre (35.2783, 9.0846) ccw projected
  arc A94 (31.5151, 6.4047) -> (31.2914, 6.1311) centre (35.7557, 2.709) ccw projected
  arc A95 (31.2914, 6.1311) -> (30.1513, 6.4711) centre (29.4123, 1.9107) ccw projected
  arc A96 (30.1513, 6.4711) -> (29.9261, 6.1118) centre (35.7557, 2.709) ccw projected
  arc A97 (29.9261, 6.1118) -> (30.7292, 5.234) centre (33.7078, 8.7656) ccw projected
  arc A98 (30.7292, 5.234) -> (30.5806, 4.9134) centre (35.7557, 2.709) ccw projected
  arc A99 (30.5806, 4.9134) -> (29.3918, 4.9591) centre (29.8101, 0.3582) ccw projected
  arc A100 (29.3918, 4.9591) -> (29.263, 4.5551) centre (35.7557, 2.709) ccw projected
  circle A101 centre (35.7557, 2.709) radius 6.75
  circle A102 centre (35.7557, 2.709) radius 7.15
  line L0 (14.7, -5.2351) -> (14.7, -14.3) projected
  line L1 (14.7, -14.3) -> (60.5, -14.3) projected
  line L2 (60.5, -14.3) -> (60.5, 13.4) projected
  line L3 (60.5, 13.4) -> (48.1174, 13.4) projected
  arc A103 (48.1174, 13.4) -> (37.9995, 13.4) centre (43.0585, 7.5289) ccw projected
  line L4 (37.9995, 13.4) -> (6.5, 13.4) projected
  line L5 (6.5, 13.4) -> (6.5, -14.3) projected
  line L6 (6.5, -14.3) -> (9.2694, -14.3) projected
  line L7 (9.2694, -14.3) -> (9.2694, -6.6578) projected
  line L8 (9.2694, -6.6578) -> (9.55, -0.45) projected
  arc A104 (20.7823, 8.7697) -> (9.55, -0.45) centre (18.95, -0.45) ccw projected
  line L9 (20.7823, 8.7697) -> (26.6956, 8.0504) projected
  arc A105 (28.6306, 5.7578) -> (26.6956, 8.0504) centre (18.95, -0.45) ccw projected
  line L10 (28.6306, 5.7578) -> (24.6721, 2.4167) projected
  arc A106 (24.6721, 2.4167) -> (14.7, -5.2351) centre (18.95, -0.45) ccw projected
  arc A107 (20.9759, -5.4556) -> (18.1049, -5.7835) centre (18.95, -0.45) ccw projected
  arc A108 (18.1049, -5.7835) -> (20.9759, -5.4556) centre (20, -9.6433) ccw projected
  arc A109 (41.3503, 0.586) -> (49.3884, 4.2041) centre (46.65, -0.45) ccw projected
  arc A110 (49.3884, 4.2041) -> (41.3503, 0.586) centre (43.0585, 7.5289) ccw projected
  point P0 (21, -14.3)
  point P1 (36.2919, 9.8389)
  point P2 (41.3938, -1.688)
  dimension "d23" = 0.4
  constraints: 1 centre point, 1 coincident, 3 other
extrude "Extrusion4" add sketch "Sketch4" along normal blind 2.6 contours A106 L10 A105 L9 A104 L8 L7 L6 L5 L4 A103 L3 L2 L1 L0
sketch "Sketch5" plane through (-21, -24.5, 14.3) normal (0, -1, 0) x (1, 0, 0)
  line L0 (12.5, 13.4) -> (6.5, 13.4) projected
  line L1 (60.5, 13.4) -> (60.5, -14.3) projected
  line L2 (6.5, 13.4) -> (60.5, 13.4)
  line L3 (60.5, 13.4) -> (60.5, -14.3)
  line L4 (60.5, -14.3) -> (6.5, -14.3)
  line L5 (6.5, -14.3) -> (6.5, 13.4)
  circle A0 centre (33.5, -7.0333) radius 8
  circle A1 centre (33.5, -7.0333) radius 8.4
  arc A2 (24.6721, 2.4167) -> (14.7, -5.2351) centre (18.95, -0.45) ccw projected
  line L6 (14.7, -5.2351) -> (14.7, -14.3) projected
  line L7 (14.7, -14.3) -> (60.5, -14.3) projected
  line L8 (60.5, -14.3) -> (60.5, 13.4) projected
  line L9 (60.5, 13.4) -> (48.1174, 13.4) projected
  arc A3 (48.1174, 13.4) -> (37.9995, 13.4) centre (43.0585, 7.5289) ccw projected
  line L10 (37.9995, 13.4) -> (6.5, 13.4) projected
  line L11 (6.5, 13.4) -> (6.5, -14.3) projected
  line L12 (6.5, -14.3) -> (9.2694, -14.3) projected
  line L13 (9.2694, -14.3) -> (9.2694, -6.6578) projected
  line L14 (9.2694, -6.6578) -> (9.55, -0.45) projected
  arc A4 (20.7823, 8.7697) -> (9.55, -0.45) centre (18.95, -0.45) ccw projected
  line L15 (20.7823, 8.7697) -> (26.6956, 8.0504) projected
  arc A5 (28.6306, 5.7578) -> (26.6956, 8.0504) centre (18.95, -0.45) ccw projected
  line L16 (28.6306, 5.7578) -> (24.6721, 2.4167) projected
  arc A6 (18.1049, -5.7835) -> (20.9759, -5.4556) centre (20, -9.6433) ccw projected
  arc A7 (20.9759, -5.4556) -> (18.1049, -5.7835) centre (18.95, -0.45) ccw projected
  arc A8 (49.3884, 4.2041) -> (36.2919, 9.8389) centre (43.0585, 7.5289) ccw projected
  arc A9 (41.3938, -1.688) -> (49.3884, 4.2041) centre (46.65, -0.45) ccw projected
  arc A10 (36.2919, 9.8389) -> (41.3938, -1.688) centre (35.7557, 2.709) ccw projected
  circle A11 centre (33.5, -7.0333) radius 1.25 projected
  arc A12 (41.4521, -7.9069) -> (40.3638, -7.4254) centre (38.8982, -12.2084) ccw projected
  arc A13 (40.3638, -7.4254) -> (40.3749, -7.0656) centre (33.5, -7.0333) ccw projected
  arc A14 (40.3749, -7.0656) -> (41.4909, -6.6522) centre (39.2074, -2.2012) ccw projected
  arc A15 (41.4909, -6.6522) -> (41.46, -6.2345) centre (33.5, -7.0333) ccw projected
  arc A16 (41.46, -6.2345) -> (40.2953, -5.9898) centre (39.8562, -10.973) ccw projected
  arc A17 (40.2953, -5.9898) -> (40.2314, -5.6355) centre (33.5, -7.0333) ccw projected
  arc A18 (40.2314, -5.6355) -> (41.2371, -4.9991) centre (38.0781, -1.1202) ccw projected
  arc A19 (41.2371, -4.9991) -> (41.12, -4.597) centre (33.5, -7.0333) ccw projected
  arc A20 (41.12, -4.597) -> (39.9299, -4.5997) centre (40.5364, -9.5654) ccw projected
  arc A21 (39.9299, -4.5997) -> (39.7937, -4.2665) centre (33.5, -7.0333) ccw projected
  arc A22 (39.7937, -4.2665) -> (40.6451, -3.4349) centre (36.7486, -0.2976) ccw projected
  arc A23 (40.6451, -3.4349) -> (40.447, -3.0659) centre (33.5, -7.0333) ccw projected
  arc A24 (40.447, -3.0659) -> (39.2834, -3.3161) centre (40.9091, -8.0471) ccw projected
  arc A25 (39.2834, -3.3161) -> (39.081, -3.0185) centre (33.5, -7.0333) ccw projected
  arc A26 (39.081, -3.0185) -> (39.7408, -2.028) centre (35.2772, 0.2307) ccw projected
  arc A27 (39.7408, -2.028) -> (39.4703, -1.7083) centre (33.5, -7.0333) ccw projected
  arc A28 (39.4703, -1.7083) -> (38.3842, -2.1948) centre (40.958, -6.4845) ccw projected
  arc A29 (38.3842, -2.1948) -> (38.1243, -1.9459) centre (33.5, -7.0333) ccw projected
  arc A30 (38.1243, -1.9459) -> (38.5638, -0.8399) centre (33.7281, 0.4414) ccw projected
  arc A31 (38.5638, -0.8399) -> (38.2327, -0.5833) centre (33.5, -7.0333) ccw projected
  arc A32 (38.2327, -0.5833) -> (37.2715, -1.2851) centre (40.6809, -4.9459) ccw projected
  arc A33 (37.2715, -1.2851) -> (36.9655, -1.0956) centre (33.5, -7.0333) ccw projected
  arc A34 (36.9655, -1.0956) -> (37.1654, 0.0776) centre (32.1691, 0.3255) ccw projected
  arc A35 (37.1654, 0.0776) -> (36.7883, 0.2597) centre (33.5, -7.0333) ccw projected
  arc A36 (36.7883, 0.2597) -> (35.994, -0.6266) centre (40.09, -3.4985) ccw projected
  arc A37 (35.994, -0.6266) -> (35.6553, -0.5048) centre (33.5, -7.0333) ccw projected
  arc A38 (35.6553, -0.5048) -> (35.6069, 0.6843) centre (30.6682, -0.112) ccw projected
  arc A39 (35.6069, 0.6843) -> (35.2001, 0.784) centre (33.5, -7.0333) ccw projected
  arc A40 (35.2001, 0.784) -> (34.6074, -0.248) centre (39.2111, -2.2056) ccw projected
  arc A41 (34.6074, -0.248) -> (34.2508, -0.1994) centre (33.5, -7.0333) ccw projected
  arc A42 (34.2508, -0.1994) -> (33.9563, 0.9537) centre (29.291, -0.852) ccw projected
  arc A43 (33.9563, 0.9537) -> (33.5377, 0.9666) centre (33.5, -7.0333) ccw projected
  arc A44 (33.5377, 0.9666) -> (33.1725, -0.1661) centre (38.0825, -1.1237) ccw projected
  arc A45 (33.1725, -0.1661) -> (32.8136, -0.1926) centre (33.5, -7.0333) ccw projected
  arc A46 (32.8136, -0.1926) -> (32.2857, 0.874) centre (28.0979, -1.8622) ccw projected
  arc A47 (32.2857, 0.874) -> (31.8736, 0.7997) centre (33.5, -7.0333) ccw projected
  arc A48 (31.8736, 0.7997) -> (31.7519, -0.3842) centre (36.7537, -0.3) ccw projected
  arc A49 (31.7519, -0.3842) -> (31.4063, -0.4848) centre (33.5, -7.0333) ccw projected
  arc A50 (31.4063, -0.4848) -> (30.6683, 0.4488) centre (27.1408, -3.0984) ccw projected
  arc A51 (30.6683, 0.4488) -> (30.2806, 0.2903) centre (33.5, -7.0333) ccw projected
  arc A52 (30.2806, 0.2903) -> (30.4077, -0.893) centre (35.2827, 0.2293) ccw projected
  arc A53 (30.4077, -0.893) -> (30.0906, -1.0632) centre (33.5, -7.0333) ccw projected
  arc A54 (30.0906, -1.0632) -> (29.1745, -0.3035) centre (26.4616, -4.5065) ccw projected
  arc A55 (29.1745, -0.3035) -> (28.8282, -0.5391) centre (33.5, -7.0333) ccw projected
  arc A56 (28.8282, -0.5391) -> (29.1986, -1.6701) centre (33.7338, 0.4413) ccw projected
  arc A57 (29.1986, -1.6701) -> (28.9238, -1.9025) centre (33.5, -7.0333) ccw projected
  arc A58 (28.9238, -1.9025) -> (27.8698, -1.3498) centre (26.0901, -6.0251) ccw projected
  arc A59 (27.8698, -1.3498) -> (27.5801, -1.6523) centre (33.5, -7.0333) ccw projected
  arc A60 (27.5801, -1.6523) -> (28.1776, -2.6816) centre (32.1746, 0.3265) ccw projected
  arc A61 (28.1776, -2.6816) -> (27.9571, -2.9661) centre (33.5, -7.0333) ccw projected
  arc A62 (27.9571, -2.9661) -> (26.8112, -2.6446) centre (26.0424, -7.5877) ccw projected
  arc A63 (26.8112, -2.6446) -> (26.5907, -3.0007) centre (33.5, -7.0333) ccw projected
  arc A64 (26.5907, -3.0007) -> (27.3891, -3.8833) centre (30.6734, -0.1099) ccw projected
  arc A65 (27.3891, -3.8833) -> (27.2326, -4.2074) centre (33.5, -7.0333) ccw projected
  arc A66 (27.2326, -4.2074) -> (26.0449, -4.1312) centre (26.3207, -9.1261) ccw projected
  arc A67 (26.0449, -4.1312) -> (25.9033, -4.5253) centre (33.5, -7.0333) ccw projected
  arc A68 (25.9033, -4.5253) -> (26.8677, -5.2226) centre (29.2957, -0.8488) ccw projected
  arc A69 (26.8677, -5.2226) -> (26.782, -5.5722) centre (33.5, -7.0333) ccw projected
  arc A70 (26.782, -5.5722) -> (25.6045, -5.7446) centre (26.9127, -10.5731) ccw projected
  arc A71 (25.6045, -5.7446) -> (25.5479, -6.1596) centre (33.5, -7.0333) ccw projected
  arc A72 (25.5479, -6.1596) -> (26.6362, -6.6411) centre (28.1018, -1.8581) ccw projected
  arc A73 (26.6362, -6.6411) -> (26.6251, -7.0009) centre (33.5, -7.0333) ccw projected
  arc A74 (26.6251, -7.0009) -> (25.5091, -7.4143) centre (27.7926, -11.8653) ccw projected
  arc A75 (25.5091, -7.4143) -> (25.54, -7.832) centre (33.5, -7.0333) ccw projected
  arc A76 (25.54, -7.832) -> (26.7047, -8.0768) centre (27.1438, -3.0935) ccw projected
  arc A77 (26.7047, -8.0768) -> (26.7686, -8.431) centre (33.5, -7.0333) ccw projected
  arc A78 (26.7686, -8.431) -> (25.7629, -9.0674) centre (28.9219, -12.9463) ccw projected
  arc A79 (25.7629, -9.0674) -> (25.88, -9.4696) centre (33.5, -7.0333) ccw projected
  arc A80 (25.88, -9.4696) -> (27.0701, -9.4668) centre (26.4636, -4.5012) ccw projected
  arc A81 (27.0701, -9.4668) -> (27.2063, -9.8) centre (33.5, -7.0333) ccw projected
  arc A82 (27.2063, -9.8) -> (26.3549, -10.6316) centre (30.2514, -13.769) ccw projected
  arc A83 (26.3549, -10.6316) -> (26.553, -11.0006) centre (33.5, -7.0333) ccw projected
  arc A84 (26.553, -11.0006) -> (27.7166, -10.7505) centre (26.0909, -6.0195) ccw projected
  arc A85 (27.7166, -10.7505) -> (27.919, -11.0481) centre (33.5, -7.0333) ccw projected
  arc A86 (27.919, -11.0481) -> (27.2592, -12.0385) centre (31.7228, -14.2972) ccw projected
  arc A87 (27.2592, -12.0385) -> (27.5297, -12.3583) centre (33.5, -7.0333) ccw projected
  arc A88 (27.5297, -12.3583) -> (28.6158, -11.8717) centre (26.042, -7.5821) ccw projected
  arc A89 (28.6158, -11.8717) -> (28.8757, -12.1207) centre (33.5, -7.0333) ccw projected
  arc A90 (28.8757, -12.1207) -> (28.4362, -13.2267) centre (33.2719, -14.508) ccw projected
  arc A91 (28.4362, -13.2267) -> (28.7673, -13.4832) centre (33.5, -7.0333) ccw projected
  arc A92 (28.7673, -13.4832) -> (29.7285, -12.7814) centre (26.3191, -9.1207) ccw projected
  arc A93 (29.7285, -12.7814) -> (30.0345, -12.9709) centre (33.5, -7.0333) ccw projected
  arc A94 (30.0345, -12.9709) -> (29.8346, -14.1441) centre (34.8309, -14.392) ccw projected
  arc A95 (29.8346, -14.1441) -> (30.2117, -14.3262) centre (33.5, -7.0333) ccw projected
  arc A96 (30.2117, -14.3262) -> (31.006, -13.44) centre (26.91, -10.5681) ccw projected
  arc A97 (31.006, -13.44) -> (31.3447, -13.5617) centre (33.5, -7.0333) ccw projected
  arc A98 (31.3447, -13.5617) -> (31.3931, -14.7508) centre (36.3318, -13.9545) ccw projected
  arc A99 (31.3931, -14.7508) -> (31.7999, -14.8505) centre (33.5, -7.0333) ccw projected
  arc A100 (31.7999, -14.8505) -> (32.3926, -13.8185) centre (27.7889, -11.861) ccw projected
  arc A101 (32.3926, -13.8185) -> (32.7492, -13.8671) centre (33.5, -7.0333) ccw projected
  arc A102 (32.7492, -13.8671) -> (33.0437, -15.0202) centre (37.709, -13.2145) ccw projected
  arc A103 (33.0437, -15.0202) -> (33.4623, -15.0332) centre (33.5, -7.0333) ccw projected
  arc A104 (33.4623, -15.0332) -> (33.8275, -13.9005) centre (28.9175, -12.9429) ccw projected
  arc A105 (33.8275, -13.9005) -> (34.1864, -13.8739) centre (33.5, -7.0333) ccw projected
  arc A106 (34.1864, -13.8739) -> (34.7143, -14.9406) centre (38.9021, -12.2043) ccw projected
  arc A107 (34.7143, -14.9406) -> (35.1264, -14.8662) centre (33.5, -7.0333) ccw projected
  arc A108 (35.1264, -14.8662) -> (35.2481, -13.6823) centre (30.2463, -13.7665) ccw projected
  arc A109 (35.2481, -13.6823) -> (35.5937, -13.5817) centre (33.5, -7.0333) ccw projected
  arc A110 (35.5937, -13.5817) -> (36.3317, -14.5153) centre (39.8592, -10.9682) ccw projected
  arc A111 (36.3317, -14.5153) -> (36.7194, -14.3569) centre (33.5, -7.0333) ccw projected
  arc A112 (36.7194, -14.3569) -> (36.5923, -13.1736) centre (31.7173, -14.2958) ccw projected
  arc A113 (36.5923, -13.1736) -> (36.9094, -13.0033) centre (33.5, -7.0333) ccw projected
  arc A114 (36.9094, -13.0033) -> (37.8255, -13.7631) centre (40.5384, -9.56) ccw projected
  arc A115 (37.8255, -13.7631) -> (38.1718, -13.5275) centre (33.5, -7.0333) ccw projected
  arc A116 (38.1718, -13.5275) -> (37.8014, -12.3965) centre (33.2662, -14.5078) ccw projected
  arc A117 (37.8014, -12.3965) -> (38.0762, -12.164) centre (33.5, -7.0333) ccw projected
  arc A118 (38.0762, -12.164) -> (39.1302, -12.7167) centre (40.9099, -8.0414) ccw projected
  arc A119 (39.1302, -12.7167) -> (39.4199, -12.4142) centre (33.5, -7.0333) ccw projected
  arc A120 (39.4199, -12.4142) -> (38.8224, -11.3849) centre (34.8254, -14.393) ccw projected
  arc A121 (38.8224, -11.3849) -> (39.0429, -11.1004) centre (33.5, -7.0333) ccw projected
  arc A122 (39.0429, -11.1004) -> (40.1888, -11.4219) centre (40.9576, -6.4788) ccw projected
  arc A123 (40.1888, -11.4219) -> (40.4093, -11.0658) centre (33.5, -7.0333) ccw projected
  arc A124 (40.4093, -11.0658) -> (39.6109, -10.1833) centre (36.3266, -13.9567) ccw projected
  arc A125 (39.6109, -10.1833) -> (39.7674, -9.8591) centre (33.5, -7.0333) ccw projected
  arc A126 (39.7674, -9.8591) -> (40.9551, -9.9353) centre (40.6793, -4.9404) ccw projected
  arc A127 (40.9551, -9.9353) -> (41.0967, -9.5412) centre (33.5, -7.0333) ccw projected
  arc A128 (41.0967, -9.5412) -> (40.1323, -8.8439) centre (37.7043, -13.2177) ccw projected
  arc A129 (40.1323, -8.8439) -> (40.218, -8.4943) centre (33.5, -7.0333) ccw projected
  arc A130 (40.218, -8.4943) -> (41.3955, -8.3219) centre (40.0873, -3.4935) ccw projected
  arc A131 (41.3955, -8.3219) -> (41.4521, -7.9069) centre (33.5, -7.0333) ccw projected
  point P0 (21, -14.3)
  point P1 (28.0205, -13.4)
  point P2 (38.9795, -13.4)
  point P3 (60.5, 13.4)
  point P4 (14.7, -14.3)
  point P5 (29.2864, -14.3)
  point P6 (29.092, 0.1172)
  point P7 (40.6022, -2.5478)
  point P8 (37.7136, -14.3)
  point P9 (37.9995, 13.4)
  point P10 (9.2694, -14.3)
  dimension "d26" = 0.4
  constraints: 8 end point, 2 parallel, 1 centre point, 1 coincident, 1 horizontal, 1 perpendicular, 3 other
extrude "Extrusion5" add sketch "Sketch5" along normal blind 2.1 contours L2 A8 A10 A1 L4 L6 A2 L16 A5 L15 A4 L14 L13 L5 L0 | A3 L2 A8 | L2 L1 L4 A1 A10 A9 A8 | L13 L14 A4 L15 A5 L16 A2 L6 L4 | A7 A6